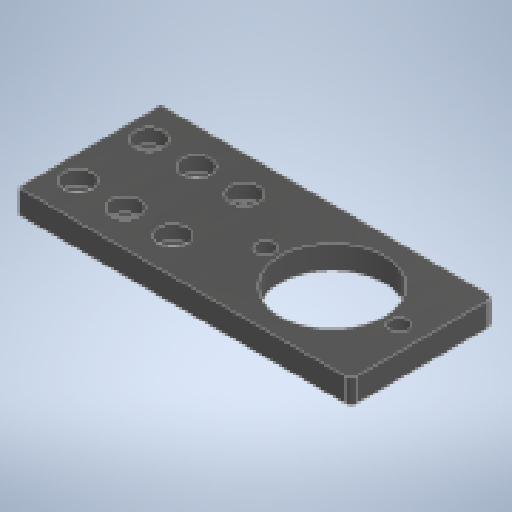
# Autodesk Inventor part: HCMUTE-CDT23-BAT_TRUC_DAN
Saved by Autodesk Inventor 2023 (Build 270158000, 158)
## iProperties
Created: 2023-11-19
Part Number: HCMUTE-CDT23-BAT_TRUC_DAN
Material: Stainless Steel
Document SubType Name: Sheet Metal
Designer: havie
Density: 8 g/cm^3
Sheet Metal Rule: Default_mm
Appearance: Dark Gray
Mass: 527.224 g
Surface Area: 202.422 cm^2
Volume: 65.903 cm^3
Author: havie
Autodesk Inventor part; units mm, degrees
ref_plane "YZ Plane" through (0, 0, 0) normal (1, 0, 0) x (0, 1, 0)
ref_plane "XZ Plane" through (0, 0, 0) normal (0, 1, 0) x (-1, 0, 0)
ref_plane "XY Plane" through (0, 0, 0) normal (0, 0, 1) x (1, 0, 0)
sketch "Sketch1" plane through (0, 0, 0) normal (0, 1, 0) x (-1, 0, 0)
  line L0 (-98, 30) -> (98, 30)
  line L1 (100, 28) -> (100, -28)
  line L2 (98, -30) -> (-98, -30)
  line L3 (-100, -28) -> (-100, 28)
  line L4 (-100, 30) -> (100, -30) construction
  line L5 (100, 30) -> (-100, -30) construction
  arc A0 (-98, 30) -> (-100, 28) centre (-98, 28) ccw
  arc A1 (100, 28) -> (98, 30) centre (98, 28) ccw
  arc A2 (98, -30) -> (100, -28) centre (98, -28) ccw
  arc A3 (-100, -28) -> (-98, -30) centre (-98, -28) ccw
  circle A4 centre (-22, 0) radius 22
  circle A5 centre (-50, 0) radius 3.75
  circle A6 centre (6, 0) radius 3.75
  circle A7 centre (30, 15) radius 3.25
  circle A8 centre (50, 15) radius 3.25
  circle A9 centre (70, 15) radius 3.25
  circle A10 centre (30, -15) radius 3.25
  circle A11 centre (50, -15) radius 3.25
  circle A12 centre (70, -15) radius 3.25
  point P0 (0, 0)
  point P1 (-100, 0)
  dimension "d0" = 60
  dimension "d1" = 200
  dimension "d2" = 2
  dimension "d3" = 44
  dimension "d4" = 56
  dimension "d5" = 28
  dimension "d6" = 7.5
  dimension "d7" = 7.5
  dimension "d8" = 50
  dimension "d9" = 6.5
  dimension "d10" = 6.5
  dimension "d11" = 6.5
  dimension "d12" = 6.5
  dimension "d13" = 6.5
  dimension "d14" = 6.5
  dimension "d15" = 15
  dimension "d16" = 30
  dimension "d17" = 30
  dimension "d18" = 20
  dimension "d19" = 20
  measures "d0" distance of L5.end L4.start
  measures "d1" distance of L4.end L5.end
  measures "d2" radius of A0
  measures "d3" diameter of A4
  measures "d4" distance of A6.centre A5.centre
  measures "d5" distance of A4.centre A5.centre
  measures "d6" diameter of A5
  measures "d7" diameter of A6
  measures "d8" distance of point (-100, 0) A5.centre
  measures "d9" diameter of A7
  measures "d10" diameter of A8
  measures "d11" diameter of A9
  measures "d12" diameter of A10
  measures "d13" diameter of A11
  measures "d14" diameter of A12
  measures "d15" distance from line of L0 A7.centre
  measures "d16" distance of A7.centre A10.centre
  measures "d17" distance from line of L1 A9.centre
  measures "d18" distance of A8.centre A9.centre
  measures "d19" distance of A7.centre A8.centre
extrude "Plate1" add sketch "Sketch1" along normal mid plane 10
sketch "Sketch2" plane through (0, 5, 0) normal (0, 1, 0) x (1, 0, 0)
  line L0 (98, -30) -> (-98, -30) projected
  line L1 (100, 30) -> (60, 30)
  line L2 (60, 30) -> (60, -30)
  line L3 (60, -30) -> (100, -30)
  line L4 (100, -30) -> (100, 30)
  line L5 (100, 28) -> (100, -28) projected
  line L6 (-98, 30) -> (98, 30) projected
  point P0 (0, 0)
  dimension "d21" = 40
  constraints: 8 end point, 2 horizontal alignment, 2 parallel, 1 horizontal, 1 perpendicular, 1 point on line, 1 vertical alignment
  measures "d21" distance between parallel lines of L4 L2
extrude "Cut1" cut sketch "Sketch2" against normal blind 10
fillet "Corner Round1" radius 2 2 edges at (60, 0, -30) (60, 0, 30)
sketch "Sketch3" plane through (0, 5, 0) normal (0, 1, 0) x (1, 0, 0)
  line L0 (-98, 30) -> (58, 30) construction
  line L1 (-100, -28) -> (-100, 28) construction
  line L2 (-100, 30) -> (-80, 30)
  line L3 (-80, 30) -> (-80, -30)
  line L4 (-80, -30) -> (-100, -30)
  line L5 (-100, -30) -> (-100, 30)
  circle A0 centre (-70, -15) radius 3.25 projected
  point P0 (0, 0)
  point P1 (-98, -30)
  dimension "d26" = 20
  constraints: 8 end point, 2 horizontal alignment, 2 parallel, 1 horizontal, 1 perpendicular, 1 vertical alignment
  measures "d26" distance between parallel lines of L3 L5
extrude "Cut2" cut sketch "Sketch3" against normal blind 10 contours L2 L3 L4 L5
sketch "Sketch4" plane through (0, 5, 0) normal (0, 1, 0) x (1, 0, 0)
  circle A0 centre (-70, 15) radius 3.25 projected
  circle A1 centre (-50, 15) radius 3.25 projected
  circle A2 centre (-30, 15) radius 3.25 projected
  circle A3 centre (-30, -15) radius 3.25 projected
  circle A4 centre (-50, -15) radius 3.25 projected
  circle A5 centre (-70, -15) radius 3.25 projected
  point P0 (0, 0)
  constraints: 6 coincident
hole "Hole1" at (-70, 5, -15) at (-50, 5, -15) at (-30, 5, -15) at (-30, 5, 15) at (-50, 5, 15) at (-70, 5, 15) direction (0, -1, 0) diameter 12 depth 6
equation "\"d7\" = d6"
equation "\"d10\" = d9"
equation "\"d11\" = d9"
equation "\"d12\" = d9"
equation "\"d13\" = d9"
equation "\"d14\" = d9"
equation "\"d22\" = Thickness"
equation "\"d27\" = Thickness"
equation "\"d20\" = Thickness"
equation "\"BendReliefDepth\" = 0.5 * Thickness"
equation "\"Thickness\" = 10"
body "Solid1"
